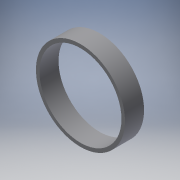
# Autodesk Inventor part: focusSpacer
Saved by Autodesk Inventor 2017 (Build 210142000, 142)
## iProperties
Created: 2016-12-19
Part Number: focusSpacer
Material: Generic
Document SubType Name: Modeling
Designer: PLTW
Density: 1 g/cm^3
Appearance: Default
Author: PLTW
Autodesk Inventor part; units mm, degrees
ref_plane "YZ Plane" through (0, 0, 0) normal (1, 0, 0) x (0, 1, 0)
ref_plane "XZ Plane" through (0, 0, 0) normal (0, 1, 0) x (-1, 0, 0)
sketch "Sketch1" plane through (0, 0, 0) normal (0, 0, 1) x (1, 0, 0)
  circle A0 centre (-5.5213, 0) radius 7.0104 projected
  circle A1 centre (-5.5213, 0) radius 5.9436 projected
  circle A2 centre (-5.5213, 0) radius 6.4516
  circle A3 centre (-5.5213, 0) radius 7.0104
  point P0 (0, 0)
  dimension "d3" = 0.508
  constraints: 2 centre point, 2 coincident, 1 concentric
  measures "d3" radial gap between concentric circles of A1 A2
ref_plane "Work Plane1" through (-12.5317, -7.0104, 2.9972) normal (0, 0, -1) x (0, 1, 0)
extrude "Extrusion1" add sketch "Sketch1" along normal up to surface (2.9972 mm away) contours A0
body "Solid1"
